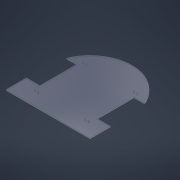
# Autodesk Inventor part: flame
Saved by Autodesk Inventor 2022 (Build 260153000, 153)
## iProperties
Created: 2021-09-22
Part Number: flame
Material: エポキシ樹脂
Document SubType Name: Modeling
Designer: shiok
Density: 1.14 g/cm^3
Appearance: 透明 - スレート 青
Author: shiok
Autodesk Inventor part; units mm, degrees
ref_plane "YZ Plane" through (0, 0, 0) normal (1, 0, 0) x (0, 1, 0)
ref_plane "XZ Plane" through (0, 0, 0) normal (0, 1, 0) x (-1, 0, 0)
ref_plane "XY Plane" through (0, 0, 0) normal (0, 0, 1) x (1, 0, 0)
sketch "スケッチ1" plane through (0, 0, 0) normal (0, 1, 0) x (-1, 0, 0)
  circle A0 centre (0, 0) radius 62.5
  line L0 (62.5, 0) -> (-62.5, 0)
  line L1 (-62.5, 0) -> (-62.5, 62.5)
  line L2 (-62.5, 62.5) -> (62.5, 62.5)
  line L3 (62.5, 62.5) -> (62.5, 0)
  point P0 (0, 62.5)
  point P1 (3.75, -60.165)
  point P2 (-3.75, -60.165)
  dimension "d41" = 125
  dimension "d70" = 60.165
  dimension "d71" = 7.5
  dimension "d72" = 3.75
  constraints: 8 end point, 2 parallel, 2 point on circle, 1 centre point, 1 coincident, 1 horizontal, 1 horizontal alignment, 1 midpoint, 1 perpendicular, 1 tangent, 1 other
  measures "d41" diameter of A0
  measures "d70" vertical distance of point (3.75, -60.165) A0.centre
  measures "d71" distance of point (-3.75, -60.165) point (3.75, -60.165)
  measures "d72" horizontal distance of A0.centre point (3.75, -60.165)
extrude "押し出し1" add sketch "スケッチ1" along normal blind 1.6
sketch "スケッチ6" plane through (0, 1.6, 0) normal (0, 1, 0) x (-1, 0, 0)
  line L0 (-35, -30) -> (-35, 42) construction
  line L1 (-35, 42) -> (-40, 42) construction
  line L2 (-40, 42) -> (-40, -30) construction
  line L3 (-35, 12) -> (-40, 12) construction
  line L4 (-42.5, 21.5) -> (-42.5, -18.5) construction
  line L5 (-35, -30) -> (-40, -30) construction
  line L6 (-42.5, 20) -> (-42.5, -20) construction
  point P0 (0, 0)
  dimension "d52" = 5
  dimension "d53" = 72
  dimension "d54" = 30
  dimension "d55" = 2.5
  dimension "d68" = 35
  dimension "d69" = 12
  constraints: 14 end point, 2 point on line, 1 horizontal, 1 parallel, 1 perpendicular
  measures "d52" distance of L1.end L0.end
  measures "d53" distance of L0.end L0.start
  measures "d54" distance between parallel lines of L1 L3
  measures "d55" distance between parallel lines of L2 L4
  measures "d68" distance from line of point (0, 0) L0
  measures "d69" distance from line of point (0, 0) L3
hole "穴3" at (35, 1.6, 42) at (40, 1.6, 42) at (40, 1.6, -30) at (35, 1.6, -30) direction (0, -1, 0) diameter 2.013 end through all thread size "M2.5x0.45" class "6H" standard "ISO Metric profile"
mirror "ミラー2" about plane through (0, 0, 0) normal (1, 0, 0) of "穴3"
sketch "スケッチ9" plane through (0, 1.6, 0) normal (0, 1, 0) x (1, 0, 0)
  line L0 (-70.8543, 23) -> (-42.5, 23)
  line L1 (-42.5, 23) -> (-42.5, -32)
  line L2 (-42.5, -32) -> (-70.8543, -32)
  line L3 (-70.8543, -32) -> (-70.8543, 23)
  line L4 (-62.5, 0) -> (-62.5, -62.5) projected
  line L5 (-62.5, -62.5) -> (62.5, -62.5) projected
  point P0 (0, 0)
  dimension "d83" = 85.5
  dimension "d84" = 55
  dimension "d85" = 20
  constraints: 8 end point, 2 parallel, 1 horizontal, 1 perpendicular
  measures "d83" distance between parallel lines of L0 L5
  measures "d84" distance between parallel lines of L0 L2
  measures "d85" distance between parallel lines of L1 L4
extrude "押し出し2" cut sketch "スケッチ9" against normal blind 10
mirror "ミラー3" about plane through (0, 0, 0) normal (1, 0, 0) of "押し出し2"
